Makita Crosscut Saw Foot (Autodesk Fusion 360 design; units mm, degrees)
Autodesk Fusion 360 part; units mm, degrees
sketch "Sketch1" plane through (0, 0, 0) normal (0, 0, 1) x (1, 0, 0)
  circle A0 centre (0, 0) radius 10
  circle A1 centre (0, 0) radius 5.9
  circle A2 centre (0, 0) radius 2.8
  circle A3 centre (0, 0) radius 1.35
  line L0 (-0.6583, 7.8026) -> (-0.6583, 5.6186)
  arc A4 (-0.6583, 5.6186) -> (0.6417, 5.6186) centre (-0.0083, 5.6186) ccw
  line L1 (0.6417, 5.6186) -> (0.6417, 7.8026)
  arc A5 (0.6417, 7.8026) -> (-0.6583, 7.8026) centre (-0.0083, 7.8026) ccw
  line L2 (-0.0083, 7.8026) -> (-0.0083, 5.6186) construction
  dimension "d1" = 20
  dimension "d2" = 11.8
  dimension "d3" = 5.6
  dimension "d4" = 2.7
  dimension "d10" = 1.3
  constraint coincident A0.centre A1.centre
  constraint concentric A2 A3
  constraint tangent L0 A4
  constraint tangent A4 L1
  constraint parallel L0 L1
  constraint tangent L1 A5
  constraint tangent L0 A5
  constraint vertical L2
  measures "d1" diameter of A0
  measures "d2" diameter of A1
  measures "d3" diameter of A2
  measures "d4" diameter of A3
  measures "d10" diameter of A4
extrude "Extrude1" add sketch "Sketch1" along normal blind 2.8 contours A0 | A1 L0 A4 L1 | A1 L0 A4 L1 | A1 L0 L1 A5 | A2
extrude "Extrude2" add sketch "Sketch1" along normal blind 9.8 contours A1 L0 A4 L1 picked at (-1.284, 4.3991)
